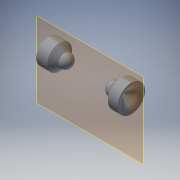
# Autodesk Inventor part: create rotation hole in pelvis
Saved by Autodesk Inventor 2019 (Build 230136000, 136)
## iProperties
Created: 2018-10-12
Part Number: create rotation hole in pelvis
Material: Generic
Document SubType Name: Modeling
Designer: HIVE
Density: 1 g/cm^3
Appearance: Default
Author: HIVE
Autodesk Inventor part; units mm, degrees
ref_plane "YZ Plane" through (0, 0, 0) normal (1, 0, 0) x (0, 1, 0)
ref_plane "XZ Plane" through (0, 0, 0) normal (0, 1, 0) x (-1, 0, 0)
ref_plane "XY Plane" through (0, 0, 0) normal (0, 0, 1) x (1, 0, 0)
ref_plane "Work Plane1" through (0, 0, 0) normal (0, 0, 1) x (1, 0, 0)
sketch "Sketch1" plane through (0, 0, 0) normal (0, 0, 1) x (1, 0, 0)
  line L0 (-49.7315, 70) -> (-40.2643, 60.5328) projected
  ellipse E0 centre (-38.9815, 70) end of major axis (-49.7315, 70) minor radius 9.5354 (-40.2643, 60.5328) -> (-28.2315, 70) ccw projected
  line L1 (-28.2315, 70) -> (-32.2315, 70) projected
  ellipse E1 centre (-38.9815, 70) end of major axis (-45.7315, 70) minor radius 5.9873 (-45.7315, 70) -> (-32.2315, 70) ccw projected
  line L2 (-45.7315, 70) -> (-49.7315, 70) projected
  line L3 (-40.2643, 60.5328) -> (-49.7315, 70) projected
  arc A0 (-60.4815, 59.25) -> (-64.8022, 50.5) centre (-49.7315, 48.5) ccw
  line L4 (-60.4815, 59.25) -> (-49.7315, 70)
  line L5 (-47.7315, 50.5) -> (-38.9815, 59.25)
  line L6 (-49.7315, 70) -> (-40.2643, 60.5328) projected
  ellipse E2 centre (-38.9815, 70) end of major axis (-49.7315, 70) minor radius 9.5354 (-40.2643, 60.5328) -> (-28.2315, 70) ccw projected
  line L7 (-28.2315, 70) -> (-32.2315, 70) projected
  ellipse E3 centre (-38.9815, 70) end of major axis (-45.7315, 70) minor radius 5.9873 (-45.7315, 70) -> (-32.2315, 70) ccw projected
  line L8 (-45.7315, 70) -> (-49.7315, 70) projected
  ellipse E4 centre (-38.9815, 70) end of major axis (-49.7315, 70) minor radius 9.5354 (-40.2643, 60.5328) -> (-28.2315, 70) ccw projected
  arc A1 (-38.9815, 59.25) -> (-28.2315, 70) centre (-38.9815, 70) ccw
  line L9 (-64.8022, 50.5) -> (-47.7315, 50.5)
  line L10 (-45.7315, 70) -> (-32.2315, 70)
  line L11 (49.7315, 70) -> (40.2643, 60.5328) projected
  line L12 (45.7315, 70) -> (49.7315, 70) projected
  ellipse E5 centre (38.9815, 70) end of major axis (45.7315, 70) minor radius 5.9873 (32.2315, 70) -> (45.7315, 70) ccw projected
  line L13 (28.2315, 70) -> (32.2315, 70) projected
  ellipse E6 centre (38.9815, 70) end of major axis (49.7315, 70) minor radius 9.5354 (28.2315, 70) -> (40.2643, 60.5328) ccw projected
  line L14 (49.7315, 70) -> (60.4815, 59.25)
  line L15 (38.9815, 59.25) -> (49.7315, 48.5)
  arc A2 (64.9343, 48.5) -> (60.4815, 59.25) centre (49.7315, 48.5) ccw
  line L16 (64.9343, 48.5) -> (49.7315, 48.5)
  line L17 (32.2315, 70) -> (45.7315, 70)
  arc A3 (28.2315, 70) -> (38.9815, 59.25) centre (38.9815, 70) ccw
  arc A4 (-60.8351, 59.6036) -> (-65.3625, 50) centre (-49.7315, 48.5) ccw
  line L18 (-65.3625, 50) -> (-47.5244, 50)
  line L19 (-47.5244, 50) -> (-38.7725, 58.7519)
  arc A5 (-38.7725, 58.7519) -> (-27.7315, 70) centre (-38.9815, 70) ccw
  arc A6 (65.4263, 48) -> (60.8351, 59.6036) centre (49.7315, 48.5) ccw
  line L20 (65.4263, 48) -> (49.5244, 48)
  line L21 (49.5244, 48) -> (38.6279, 58.8964)
  line L22 (38.9815, 70) -> (27.8779, 70.3536) construction
  line L23 (38.9815, 70) -> (38.6279, 58.8964) construction
  line L24 (-19.398, 70) -> (-4.8831, 70)
  line L25 (-49.7315, 70) -> (-50.4386, 70)
  line L26 (28.2315, 70) -> (27.8723, 70)
  line L27 (49.7315, 70) -> (50.4386, 70)
  line L28 (-50.4386, 70) -> (-60.8351, 59.6036)
  line L29 (-28.2315, 70) -> (-27.7315, 70)
  arc A7 (27.8723, 70) -> (38.6279, 58.8964) centre (38.9815, 70) ccw
  line L30 (50.4386, 70) -> (60.8351, 59.6036)
  point P0 (0, 0)
  dimension "d5" = 90
  constraints: 42 end point, 16 point on circle, 8 centre point, 7 horizontal, 3 coincident, 2 point on line, 1 collinear, 27 other
  measures "d5" angle of L22 L23
revolve "Revolution3" add sketch "Sketch1" angle 198 about axis through (-19.398, 70, 0) along (-1, 0, 0)
body "Solid3"
